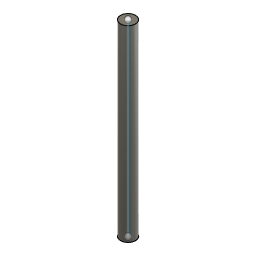
Pendule (Autodesk Fusion 360 design; units mm, degrees)
Autodesk Fusion 360 part; units mm, degrees
sketch "Ligne 3D" plane through (0, 0, 0) normal (1, 0, 0) x (0, 0, -1)
  line L0 (-2.6562, 0.8961) -> (-2.6562, 150.8961)
ref_plane "WorkPlane1" through (0, 0.8961, 2.6562) normal (0, 1, 0) x (-1, 0, 0)
sketch "Section" plane through (0, 0.8961, 2.6562) normal (0, 1, 0) x (1, 0, 0)
  circle A0 centre (0, 0) radius 6
  dimension "d3" = 12
  constraint coincident A0.centre origin
  measures "d3" diameter of A0
sweep "Sweep1" add profiles "Section" path "Ligne 3D" along L0 section 1
